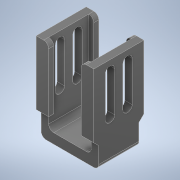
# Autodesk Inventor part: magnetsupport
Saved by Autodesk Inventor 2022 (Build 260153000, 153)
## iProperties
Created: 2022-08-13
Part Number: magnetsupport
Material: Genérico
Document SubType Name: Modeling
Designer: JK
Density: 1 g/cm^3
Appearance: Suave - Negro
Author: JK
Autodesk Inventor part; units mm, degrees
ref_plane "YZ Plane" through (0, 0, 0) normal (1, 0, 0) x (0, 1, 0)
ref_plane "XZ Plane" through (0, 0, 0) normal (0, 1, 0) x (-1, 0, 0)
ref_plane "XY Plane" through (0, 0, 0) normal (0, 0, 1) x (1, 0, 0)
sketch "Boceto1" plane through (0, 0, 0) normal (0, 1, 0) x (-1, 0, 0)
  circle A0 centre (0, 0) radius 2.25
  line L0 (-8.5, 8) -> (8.5, 8)
  line L1 (8.5, 8) -> (8.5, -8)
  line L2 (8.5, -8) -> (-8.5, -8)
  line L3 (-8.5, -8) -> (-8.5, 8)
  line L4 (-8.5, 8) -> (8.5, -8) construction
  line L5 (8.5, 8) -> (-8.5, -8) construction
  dimension "d0" = 4.5
  dimension "d1" = 17
  dimension "d2" = 16
  constraints: 12 end point, 2 midpoint, 2 parallel, 1 centre point, 1 coincident, 1 horizontal, 1 perpendicular
  measures "d0" diameter of A0
  measures "d1" distance of L1.end L2.end
  measures "d2" distance of L0.end L1.end
extrude "Extrusión1" add sketch "Boceto1" along normal blind 4
sketch "Boceto3" plane through (0, 0, 0) normal (0, -1, 0) x (1, 0, 0)
  line L0 (11.5, 8) -> (-11.5, 8)
  line L1 (-11.5, 8) -> (-11.5, -8)
  line L2 (-11.5, -8) -> (11.5, -8)
  line L3 (11.5, -8) -> (11.5, 8)
  circle A0 centre (0, 0) radius 2.25 projected
  line L4 (11.5, 8) -> (-11.5, -8) construction
  line L5 (-11.5, 8) -> (11.5, -8) construction
  line L6 (8.5, -8) -> (-8.5, -8) projected
  line L7 (8.5, 8) -> (8.5, -8) projected
  line L8 (8.5, -8) -> (-8.5, -8) projected
  line L9 (8.5, 8) -> (8.5, -8) projected
  line L10 (-8.5, 8) -> (8.5, 8) projected
  line L11 (-8.5, -8) -> (-8.5, 8) projected
  circle A1 centre (0, 0) radius 2.25 projected
  point P0 (8.5, -8)
  point P1 (-8.5, -8)
  point P2 (-8.5, 8)
  dimension "d8" = 3
  constraints: 12 end point, 2 midpoint, 2 parallel, 1 collinear, 1 horizontal, 1 perpendicular
  measures "d8" distance between parallel lines of L7 L3
extrude "Extrusión3" add sketch "Boceto3" against normal blind 36 contours L3 L2 L7 L0 | L11 L2 L1 L0
sketch "Boceto4" plane through (11.5, 0, 8) normal (1, 0, 0) x (0, 0, -1)
  circle A0 centre (4.5, 16) radius 1.85
  circle A1 centre (11.5, 16) radius 1.85
  line L0 (0, 36) -> (16, 36) projected
  line L1 (0, 0) -> (0, 36) projected
  line L2 (2.65, 36) -> (6.35, 36)
  line L3 (6.35, 36) -> (6.35, 16)
  line L4 (6.35, 16) -> (2.65, 16)
  line L5 (2.65, 16) -> (2.65, 36)
  line L6 (9.65, 36) -> (13.35, 36)
  line L7 (13.35, 36) -> (13.35, 16)
  line L8 (13.35, 16) -> (9.65, 16)
  line L9 (9.65, 16) -> (9.65, 36)
  circle A2 centre (4.5, 32) radius 1.85
  circle A3 centre (11.5, 32) radius 1.85
  point P0 (8, 0)
  point P1 (9.65, 36)
  point P2 (9.65, 16)
  point P3 (9.65, 32)
  point P4 (13.35, 32)
  point P5 (2.65, 32)
  point P6 (6.35, 32)
  dimension "d11" = 20
  dimension "d12" = 3.7
  dimension "d14" = 7
  dimension "d18" = 4.5
  dimension "d28" = 4
  dimension "d29" = 4
  constraints: 16 end point, 6 tangent, 4 parallel, 3 centre point, 2 collinear, 2 horizontal, 2 perpendicular, 2 vertical, 1 horizontal alignment, 1 point on line, 4 other
  measures "d11" distance from line of L0 A1.centre
  measures "d12" diameter of A1
  measures "d14" distance of A1.centre point (4.5, 16)
  measures "d18" distance from line of L1 point (4.5, 16)
  measures "d28" distance from line of L0 A2.centre
  measures "d29" distance from line of L6 A3.centre
extrude "Extrusión4" cut sketch "Boceto4" against normal through all contours L4 A0 | A0 L5 A2 L3 | A0 L4 | A2 | L8 A1 | A1 L9 A3 L7 | A1 L8 | A3
fillet "Empalme1" radius 2 2 edges at (-11.5, 0, 0) (11.5, 0, 0)
sketch "Boceto6" plane through (0, 0, 0) normal (0, -1, 0) x (1, 0, 0)
  circle A0 centre (0, 0) radius 5
  dimension "d24" = 10
  constraints: 1 centre point, 1 coincident
  measures "d24" diameter of A0
extrude "Extrusión6" [suppressed]
fillet "Empalme2" radius 2 2 edges at (-8.5, 4, 0) (8.5, 4, 0)
sketch "Boceto8" plane through (0, 36, 0) normal (0, 1, 0) x (1, 0, 0)
  line L0 (-11.5, -10) -> (11.5, -10)
  line L1 (11.5, -10) -> (11.5, 10)
  line L2 (11.5, 10) -> (-11.5, 10)
  line L3 (-11.5, 10) -> (-11.5, -10)
  line L4 (-11.5, -10) -> (11.5, 10) construction
  line L5 (11.5, -10) -> (-11.5, 10) construction
  line L6 (11.5, -8) -> (11.5, 8) projected
  line L7 (-8.5, 8) -> (-11.5, 8) projected
  line L8 (-6.5, -10) -> (6.5, -10)
  line L9 (6.5, -10) -> (6.5, 10)
  line L10 (6.5, 10) -> (-6.5, 10)
  line L11 (-6.5, 10) -> (-6.5, -10)
  circle A0 centre (0, 0) radius 2.25 projected
  line L12 (-6.5, -10) -> (6.5, 10) construction
  line L13 (6.5, -10) -> (-6.5, 10) construction
  line L14 (8.5, 8) -> (8.5, -8) projected
  line L15 (11.5, -8) -> (-11.5, -8)
  line L16 (-11.5, -8) -> (-11.5, 8)
  line L17 (-11.5, 8) -> (11.5, 8)
  line L18 (11.5, 8) -> (11.5, -8)
  line L19 (11.5, -8) -> (-11.5, 8) construction
  line L20 (-11.5, -8) -> (11.5, 8) construction
  point P0 (-6.5, 8)
  point P1 (11.5, 8)
  point P2 (6.5, 8)
  point P3 (6.5, -8)
  point P4 (11.5, -8)
  point P5 (-6.5, -8)
  point P6 (-11.5, -8)
  point P7 (-6.5, -10)
  dimension "d30" = 2
  dimension "d31" = 2
  constraints: 36 end point, 6 midpoint, 6 parallel, 3 horizontal, 3 perpendicular, 1 collinear, 1 point on line
  measures "d30" distance between parallel lines of L2 L7
  measures "d31" distance between parallel lines of L9 L14
extrude "Extrusión7" add sketch "Boceto8" against normal blind 25.5 contours L3 L15 L11 L0 | L9 L15 L1 L0 | L3 L2 L11 L17 L7 | L9 L2 L1 L17
chamfer "Chaflán1" distance 2 angle 45 4 edges at (10, 10.5, 8) (-10, 10.5, 8) (10, 10.5, -8) (-10, 10.5, -8)
fillet "Empalme3" radius 2 6 edges at (-6.5, 10.5, -9) (6.5, 10.5, -9) (6.5, 36, -9) (-6.5, 36, -9) (-6.5, 36, 9) (6.5, 36, 9)
sketch "Boceto5" plane through (-11.5, 16, 5.35) normal (-1, 0, 0) x (0, 0, 1)
  arc A0 (-10.7, 0) -> (-7, 0) centre (-8.85, 0) ccw projected
  circle A1 centre (-8.85, 0) radius 2.85
  arc A2 (-3.7, 0) -> (0, 0) centre (-1.85, 0) ccw projected
  circle A3 centre (-1.85, 0) radius 2.85
  line L0 (-11.7, 0) -> (-6, 0)
  line L1 (-6, 0) -> (-6, 8.628)
  line L2 (-6, 8.628) -> (-11.7, 8.628)
  line L3 (-11.7, 8.628) -> (-11.7, 0)
  line L4 (-4.7, 0) -> (1, 0)
  line L5 (1, 0) -> (1, 8.628)
  line L6 (1, 8.628) -> (-4.7, 8.628)
  line L7 (-4.7, 8.628) -> (-4.7, 0)
  line L8 (-8.85, 3.2909) -> (-6, 1.6454)
  line L9 (-6, 1.6454) -> (-6, -1.6454)
  line L10 (-6, -1.6454) -> (-8.85, -3.2909)
  line L11 (-8.85, -3.2909) -> (-11.7, -1.6454)
  line L12 (-11.7, -1.6454) -> (-11.7, 1.6454)
  line L13 (-11.7, 1.6454) -> (-8.85, 3.2909)
  line L14 (-1.85, 3.2909) -> (1, 1.6454)
  line L15 (1, 1.6454) -> (1, -1.6454)
  line L16 (1, -1.6454) -> (-1.85, -3.2909)
  line L17 (-1.85, -3.2909) -> (-4.7, -1.6454)
  line L18 (-4.7, -1.6454) -> (-4.7, 1.6454)
  line L19 (-4.7, 1.6454) -> (-1.85, 3.2909)
  point P0 (-5.35, -16)
  point P1 (0, 0)
  point P2 (-3.5, 0)
  point P3 (1.1, 0)
  point P4 (-5.9, 0)
  point P5 (-7, 0)
  point P6 (-10.5, 0)
  point P7 (-7.325, -2.4682)
  point P8 (-5.9, 0)
  point P9 (-10.175, -2.4682)
  point P10 (-11.6, 0)
  point P11 (-4.6, 0)
  point P12 (-3.175, -2.4682)
  point P13 (-0.325, -2.4682)
  point P14 (1.1, 0)
  dimension "d20" = 5.7
  dimension "d21" = 5.7
  constraints: 40 end point, 6 vertical, 4 coincident, 4 parallel, 2 horizontal, 2 perpendicular, 2 vertical alignment, 1 point on line, 32 other
